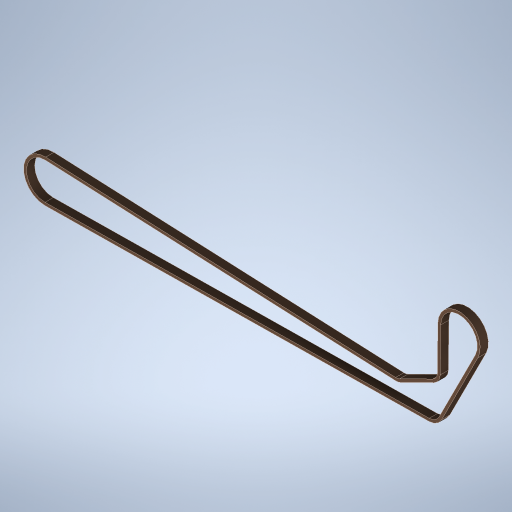
# Autodesk Inventor part: timingbelt
Saved by Autodesk Inventor 2024 (Build 280153000, 153)
## iProperties
Created: 2025-02-15
Part Number: timingbelt
Material: 一般
Document SubType Name: Modeling
Designer: tanoue_kota
Density: 1 g/cm^3
Appearance: ブロンズ - サテン
Mass: 42.8494 g
Surface Area: 337.028 cm^2
Volume: 42.8494 cm^3
Author: tanoue_kota
Autodesk Inventor part; units mm, degrees
ref_plane "YZ Plane" through (0, 0, 0) normal (1, 0, 0) x (0, 1, 0)
ref_plane "XZ Plane" through (0, 0, 0) normal (0, 1, 0) x (-1, 0, 0)
ref_plane "XY Plane" through (0, 0, 0) normal (0, 0, 1) x (1, 0, 0)
sketch "スケッチ1" plane through (0, 0, 0) normal (0, 0, 1) x (1, 0, 0)
  circle A0 centre (0, 0) radius 24.669
  line L0 (0, 0) -> (413, 0)
  line L1 (413, 0) -> (413, 89.255)
  line L2 (413, 0) -> (0, 0)
  line L3 (0, 0) -> (0, -22.279)
  line L4 (413, -7.7398) -> (413, 0)
  line L5 (0, 0) -> (0, 22.279)
  line L6 (413, 7.7398) -> (413, 0)
  circle A1 centre (425.85, 16.3792) radius 10
  circle A2 centre (502.2492, 88.554) radius 24.669
  circle A3 centre (466, -2.5437) radius 15.9155
  arc A4 (1.1659, 25.6625) -> (13.7874, 21.6756) centre (0, 0) ccw
  arc A5 (482.669, 0.449) -> (481.1136, -10.185) centre (466, -2.5437) ccw
  circle A6 centre (502.2492, 88.554) radius 25.689
  line L7 (1.1659, 25.6625) -> (425.3961, 6.3895)
  line L8 (525.1747, 76.9632) -> (481.1136, -10.185)
  line L9 (466.2257, -19.4777) -> (0.3423, -25.6867)
  circle A7 centre (0, 0) radius 22.279
  circle A8 centre (466, -2.5437) radius 13.5255
  circle A9 centre (502.2492, 88.554) radius 22.279
  circle A10 centre (425.85, 16.3792) radius 13.41
  line L10 (-9.5707, 22.7368) -> (425.2414, 2.983)
  line L11 (0.2969, -22.277) -> (466.1802, -16.068)
  line L12 (522.1316, 78.5018) -> (516.361, 67.0881)
  line L13 (516.361, 67.0881) -> (478.0705, -8.6464)
  circle A11 centre (466.033, 36.222) radius 10
  circle A12 centre (466.033, 36.222) radius 13.41
  line L14 (430.2776, 7.4129) -> (470.4607, 27.2556)
  line L15 (431.7875, 4.3553) -> (471.9705, 24.1981)
  line L16 (476.0325, 36.1216) -> (476.5615, 88.8119)
  line L17 (479.4423, 36.0874) -> (479.9714, 88.7777)
  line L18 (413, 89.255) -> (466, -2.5437)
  line L19 (466.033, 36.222) -> (413, 89.255)
  line L20 (425.85, 16.3792) -> (413, 89.255)
  line L21 (413, -7.7398) -> (469, -7.7398)
  line L22 (469, -7.7398) -> (466, -2.5437)
  line L23 (466, -2.5437) -> (457, -7.7398)
  line L24 (413, 89.255) -> (502.2492, 88.554)
  point P0 (1.0111, 22.2561)
  point P1 (457.5323, 12.1229)
  point P2 (453.6018, 18.9306)
  dimension "d0" = 49.338
  dimension "d1" = 413
  dimension "d2" = 89.255
  dimension "d6" = 20
  dimension "d8" = 49.338
  dimension "d10" = 31.831
  dimension "d11" = 1.02
  dimension "d12" = 1.02
  dimension "d14" = 2.39
  dimension "d15" = 2.39
  dimension "d17" = 3.41
  dimension "d22" = 20
  dimension "d23" = 3.41
  dimension "d31" = 75
  dimension "d32" = 15
  dimension "d36" = 2.39
  dimension "d37" = 10
  dimension "d38" = 74
  dimension "d40" = 1.02
  dimension "d41" = 89.252
  dimension "d43" = 30
  dimension "d45" = 6
  dimension "d46" = 106
  dimension "d47" = 89.55
  constraints: 50 end point, 23 point on circle, 20 tangent, 12 centre point, 3 coincident, 3 horizontal, 3 parallel, 3 point on line, 2 perpendicular, 2 symmetric about line, 1 collinear, 1 vertical, 3 other
  measures "d1" distance of L0.start L0.end
  measures "d2" distance of L0.end L1.end
  measures "d6" diameter of A1
  measures "d8" diameter of A2
  measures "d10" diameter of A3
  measures "d12" radial gap between concentric circles of A3 A5
  measures "d15" radial gap between concentric circles of A3 A8
  measures "d17" radial gap between concentric circles of A1 A10
  measures "d22" diameter of A11
  measures "d23" radial gap between concentric circles of A11 A12
  measures "d31" distance of L19.start L18.start
  measures "d32" angle of L18 L19
  measures "d36" radial gap between concentric circles of A9 A2
  measures "d37" angle of L1 L20
  measures "d38" distance of L20.start L18.start
  measures "d40" radial gap between concentric circles of A2 A6
  measures "d41" distance of L24.end L18.start
  measures "d43" angle of L1 L18
  measures "d45" distance from line of L21.end L23
  measures "d46" distance of L18.start L18.end
  measures "d47" angle of L1 L24
extrude "押し出し1" add sketch "スケッチ1" along normal blind 10 contours L10 A0 | A0 L11 A4 L7 L1 L10 | A0 L10 A7 L11 | L11 A5 L9 A4 | L1 L7 A10 L10 | L11 A3 L13 A6 L8 A5 | A10 L7 A1 L14 | L11 A8 L13 A3 | A10 L14 L18 L15 | L18 L14 A12 L15 | A6 L12 A2 L24 | A12 L14 A11 L16 | L17 A12 L16 A6 | A6 L24 A2 L17 | L12 A9 L24 A2 | A2 L24 L17
